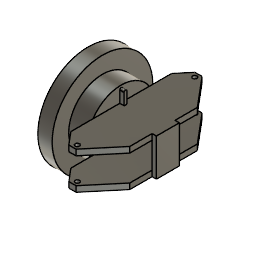
Jaw 6 (End Effector Mount) (Autodesk Fusion 360 design; units mm, degrees)
part number: 2026-06-21-13-07-49-301
Autodesk Fusion 360 part; units mm, degrees
sketch "Sketch1" plane through (0, 0, 0) normal (1, 0, 0) x (0, 1, 0)
  circle A0 centre (0, 0) radius 35
  dimension "d1" = 70
  constraint coincident A0.centre origin
  measures "d1" diameter of A0
extrude "Extrude1" add sketch "Sketch1" along normal blind 10
sketch "Sketch2" plane through (10, 0, 0) normal (1, 0, 0) x (0, 1, 0)
  circle A0 centre (0, 0) radius 35
  circle A1 centre (0, 0) radius 23.5
  dimension "d4" = 47
  constraint coincident A0.centre A1.centre
  measures "d4" diameter of A1
extrude "Extrude2" add sketch "Sketch2" along normal blind 13 contours A1
ref_plane "WorkPlane1" through (0, 0, 13) normal (0, 0, 1) x (1, 0, 0)
sketch "Sketch3" plane through (0, 0, 13) normal (0, 0, 1) x (1, 0, 0)
  line L0 (23, 0) -> (23, -35)
  line L1 (23, -35) -> (23, -45)
  line L2 (23, -35) -> (30.3921, -43.8095)
  line L3 (30.3921, -43.8095) -> (35.3921, -43.8095)
  line L4 (23, 0) -> (60, 0)
  line L5 (23, -23.5) -> (67, -23.5)
  line L6 (35.3921, -43.8095) -> (52.4338, -23.5)
  line L7 (35.3921, -43.8095) -> (47, -43.8095)
  line L8 (52.4338, -23.5) -> (52.4338, 0)
  line L9 (23, 0) -> (23, 35)
  line L10 (23, 35) -> (30.3921, 43.8095)
  line L11 (30.3921, 43.8095) -> (35.3921, 43.8095)
  line L12 (35.3921, 43.8095) -> (52.4338, 23.5)
  line L13 (52.4338, 23.5) -> (52.4338, 0)
  dimension "d8" = 35
  dimension "d9" = 10
  dimension "d10" = 11.5
  dimension "d11" = 40
  dimension "d12" = 5
  dimension "d13" = 50
  constraint vertical L0
  constraint parallel L0 L1
  constraint horizontal L3
  constraint perpendicular L0 L4
  constraint coincident L0 L5.start
  constraint perpendicular L0 L5
  constraint coincident L5 L6.end
  constraint parallel L3 L7
  constraint coincident L4 L8.end
  constraint perpendicular L4 L8
  constraint symmetric L0.start L4 L9.start
  constraint symmetric L0.end L4 L9.end
  constraint symmetric L2.end L4 L10.end
  constraint symmetric L3.end L4 L11.end
  constraint symmetric L4 L6.end L12.end
  constraint symmetric L4 L8.end L13.end
  measures "d8" distance of L0.start L0.end
  measures "d9" distance of L0.end L1.end
  measures "d10" distance of L0.end L2.end
  measures "d11" angle of L1 L2
  measures "d12" distance of L2.end L3.end
  measures "d13" angle of L6 L7
extrude "Extrude3" add sketch "Sketch3" against normal blind 4
sketch "Sketch4" plane through (0, 0, 13) normal (0, 0, 1) x (-1, 0, 0)
  line L0 (-23, -35) -> (-23, -19.5768)
  line L1 (-23, -19.5768) -> (-23, 19.5768)
  line L2 (-23, 19.5768) -> (-23, 35)
  line L3 (-23, 35) -> (-30.3921, 43.8095)
  line L4 (-30.3921, 43.8095) -> (-35.3921, 43.8095)
  line L5 (-35.3921, 43.8095) -> (-52.4338, 23.5)
  line L6 (-52.4338, 23.5) -> (-52.4338, -23.5)
  line L7 (-52.4338, -23.5) -> (-35.3921, -43.8095)
  line L8 (-35.3921, -43.8095) -> (-30.3921, -43.8095)
  line L9 (-30.3921, -43.8095) -> (-23, -35)
  line L10 (-33.3297, 43.8095) -> (-33.3297, 40.8095)
  circle A0 centre (-33.3297, 40.8095) radius 1.5
  dimension "d16" = 3
  dimension "d17" = 3
  constraint coincident L4 L10.start
  constraint perpendicular L4 L10
  constraint coincident L10.end A0.centre
  measures "d16" distance of L10.start L10.end
  measures "d17" diameter of A0
extrude "Extrude4" cut sketch "Sketch4" against normal blind 8 contours A0
mirror "Mirror1" about plane through (0, 0, 0) normal (0, 1, 0) of "Extrude4"
mirror "Mirror2" about plane through (0, 0, 0) normal (0, 0, 1) of "Extrude3", "Extrude4", "Mirror1"
sketch "Sketch5" plane through (23, 0, 0) normal (1, 0, 0) x (0, 1, 0)
  line L0 (-19.5768, 13) -> (19.5768, 13)
  arc A0 (19.5768, 13) -> (-19.5768, 13) centre (0, 0) ccw
  line L1 (0, 13) -> (0, 23.5)
  line L2 (0, 13) -> (-1, 13)
  line L3 (-1, 13) -> (-1, 22)
  line L4 (-1, 22) -> (1, 22)
  line L5 (1, 22) -> (1, 13)
  dimension "d24" = 1
  dimension "d25" = 9
  dimension "d26" = 2
  dimension "d27" = 9
  constraint midpoint L0 L1.start
  constraint midpoint A0 L1.end
  constraint perpendicular L1 L2
  constraint perpendicular L2 L3
  constraint perpendicular L1 L4
  constraint perpendicular L4 L5
  measures "d24" distance of L1.start L2.end
  measures "d25" distance of L2.end L3.end
  measures "d26" distance of L3.end L4.end
  measures "d27" distance of L4.end L5.end
extrude "Extrude5" add sketch "Sketch5" along normal blind 3 contours L0 L1 L2 L3 L4 | L0 L1 L4 L5
fillet "Fillet1" radius 1 2 edges at (24.5, 1, 22) (24.5, -1, 22)
mirror "Mirror3" about plane through (0, 0, 0) normal (0, 0, 1) of "Extrude5", "Fillet1"
sketch "Sketch6" plane through (52.4338, 0, 0) normal (1, 0, 0) x (0, 1, 0)
  line L0 (23.5, 13) -> (-23.5, 13)
  line L1 (-23.5, 13) -> (-23.5, 9)
  line L2 (-23.5, 9) -> (23.5, 9)
  line L3 (23.5, 9) -> (23.5, 13)
  line L4 (8, -13) -> (-8, -13)
  line L5 (-8, -13) -> (-8, 13)
  line L6 (-8, 13) -> (8, 13)
  line L7 (8, 13) -> (8, -13)
  line L8 (8, -13) -> (-8, 13) construction
  line L9 (-8, -13) -> (8, 13) construction
  constraint horizontal L4
  constraint perpendicular L4 L5
  constraint parallel L4 L6
  constraint parallel L5 L7
  constraint coincident L8 origin
  constraint coincident L9 origin
extrude "Extrude6" add sketch "Sketch6" along normal blind 3 contours L0 L2 L5 L6 L7 | L2 L4 L5 L7
sketch "Sketch7" plane through (0, 0, 0) normal (-1, 0, 0) x (0, -1, 0)
  circle A0 centre (0, 0) radius 35
  circle A1 centre (0, 0) radius 10
  dimension "d36" = 20
  constraint coincident A0.centre A1.centre
  measures "d36" diameter of A1
extrude "Extrude7" cut sketch "Sketch7" against normal blind 10 contours A1
